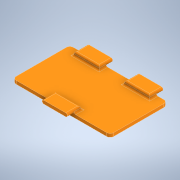
# Autodesk Inventor part: BatteryPlate
Saved by Autodesk Inventor 2021 (Build 250183000, 183)
## iProperties
Created: 2021-05-13
Part Number: BatteryPlate
Material: Generic
Document SubType Name: Modeling
Designer: ermoz
Density: 1 g/cm^3
Appearance: Default
Author: ermoz
Autodesk Inventor part; units mm, degrees
ref_plane "YZ Plane" through (0, 0, 0) normal (1, 0, 0) x (0, 1, 0)
ref_plane "XZ Plane" through (0, 0, 0) normal (0, 1, 0) x (-1, 0, 0)
ref_plane "XY Plane" through (0, 0, 0) normal (0, 0, 1) x (1, 0, 0)
sketch "Sketch1" plane through (0, 0, 0) normal (0, 1, 0) x (-1, 0, 0)
  line L0 (-29, -17) -> (29, -17)
  line L1 (29, -17) -> (29, 17)
  line L2 (29, 17) -> (-29, 17)
  line L3 (-29, 17) -> (-29, -17)
  line L4 (-29, -17) -> (29, 17) construction
  line L5 (29, -17) -> (-29, 17) construction
  point P0 (0, 0)
  dimension "d0" = 34
  dimension "d1" = 58
  constraints: 12 end point, 2 midpoint, 2 parallel, 1 horizontal, 1 perpendicular
  measures "d0" distance of L0.end L1.end
  measures "d1" distance of L1.end L2.end
extrude "Extrusion1" add sketch "Sketch1" along normal blind 2
fillet "Fillet1" radius 2 4 edges at (29, 1, 17) (29, 1, -17) (-29, 1, -17) (-29, 1, 17)
sketch "Sketch3" plane through (0, 2, 0) normal (0, 1, 0) x (1, 0, 0)
  line L0 (-22.5, 21) -> (-7.5, 21)
  line L1 (-7.5, 21) -> (-7.5, 13)
  line L2 (-7.5, 13) -> (-22.5, 13)
  line L3 (-22.5, 13) -> (-22.5, 21)
  line L4 (27, 17) -> (-27, 17) projected
  line L5 (-22.5, 21) -> (-7.5, 13) construction
  line L6 (-7.5, 21) -> (-22.5, 13) construction
  line L7 (22.5, 21) -> (7.5, 21)
  line L8 (7.5, 21) -> (7.5, 13)
  line L9 (7.5, 13) -> (22.5, 13)
  line L10 (22.5, 13) -> (22.5, 21)
  line L11 (22.5, 21) -> (7.5, 13) construction
  line L12 (7.5, 21) -> (22.5, 13) construction
  line L13 (-7.5, -13) -> (7.5, -13)
  line L14 (7.5, -13) -> (7.5, -21)
  line L15 (7.5, -21) -> (-7.5, -21)
  line L16 (-7.5, -21) -> (-7.5, -13)
  line L17 (-27, -17) -> (27, -17) projected
  line L18 (-7.5, -13) -> (7.5, -21) construction
  line L19 (7.5, -13) -> (-7.5, -21) construction
  point P0 (0, 0)
  point P1 (-15, 17)
  point P2 (15, 17)
  point P3 (0, -17)
  dimension "d9" = 15
  dimension "d10" = 8
  dimension "d11" = 15
  dimension "d12" = 15
  dimension "d13" = 8
  dimension "d14" = 15
  dimension "d15" = 15
  dimension "d16" = 8
  constraints: 36 end point, 7 midpoint, 6 parallel, 3 horizontal, 3 perpendicular, 2 point on line
  measures "d9" distance of L1.end L2.end
  measures "d10" distance of L0.end L1.end
  measures "d11" horizontal distance of point (0, 0) point (-15, 17)
  measures "d12" distance of L9.end L8.end
  measures "d13" distance of L7.end L8.end
  measures "d14" horizontal distance of point (0, 0) point (15, 17)
  measures "d15" distance of L14.end L15.end
  measures "d16" distance of L13.end L14.end
extrude "Extrusion3" add sketch "Sketch3" along normal blind 2
fillet "Fillet2" radius 1 24 edges at (7.5, 2, 15) (7.5, 4, 17) (0, 2, 13) (0, 4, 13) (-7.5, 2, 15) (-7.5, 4, 17) (-7.5, 2, 19) (7.5, 2, 19) (-22.5, 2, -15) (-22.5, 4, -17) (-15, 2, -13) (-15, 4, -13) (-7.5, 2, -15) (-7.5, 4, -17) (-22.5, 2, -19) (-7.5, 2, -19) (22.5, 2, -19) (22.5, 4, -17) (22.5, 2, -15) (15, 2, -13) (15, 4, -13) (7.5, 2, -15) (7.5, 4, -17) (7.5, 2, -19)
body "Solid1"
